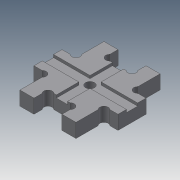
# Autodesk Inventor part: piece_1
Saved by Autodesk Inventor 2015 (Build 190159000, 159)
## iProperties
Created: 2017-11-05
Part Number: piece_1
Material: 一般
Document SubType Name: Modeling
Designer: tasuku
Density: 1 g/cm^3
Appearance: 既定
Author: tasuku
Autodesk Inventor part; units mm, degrees
ref_plane "YZ Plane" through (0, 0, 0) normal (1, 0, 0) x (0, 1, 0)
ref_plane "XZ Plane" through (0, 0, 0) normal (0, 1, 0) x (-1, 0, 0)
ref_plane "XY Plane" through (0, 0, 0) normal (0, 0, 1) x (1, 0, 0)
sketch "スケッチ1" plane through (0, 0, 0) normal (0, 0, 1) x (1, 0, 0)
  line L0 (-15, -15) -> (15, -15)
  line L1 (15, -15) -> (15, 15)
  line L2 (15, 15) -> (-15, 15)
  line L3 (-15, 15) -> (-15, -15)
  line L4 (-15, -15) -> (15, 15) construction
  line L5 (15, -15) -> (-15, 15) construction
  point P0 (0, 0)
  dimension "d2" = 30
  dimension "d3" = 30
  constraints: 12 end point, 2 midpoint, 2 parallel, 1 horizontal, 1 perpendicular
  measures "d2" distance of L1.end L2.end
  measures "d3" distance of L0.end L1.end
extrude "押し出し1" add sketch "スケッチ1" along normal blind 5
sketch "スケッチ2" plane through (0, 0, 5) normal (0, 0, 1) x (1, 0, 0)
  line L0 (-15, 15) -> (-10, 15)
  line L1 (-10, 15) -> (-10, 5)
  line L2 (-10, 5) -> (-15, 5)
  line L3 (-15, 5) -> (-15, 15)
  line L4 (-15, -15) -> (-10, -15)
  line L5 (-10, -15) -> (-10, -5)
  line L6 (-10, -5) -> (-15, -5)
  line L7 (-15, -5) -> (-15, -15)
  line L8 (15, 15) -> (-15, 15) projected
  line L9 (10, 15) -> (15, 15)
  line L10 (15, 15) -> (15, 5)
  line L11 (15, 5) -> (10, 5)
  line L12 (10, 5) -> (10, 15)
  line L13 (15, -15) -> (10, -15)
  line L14 (10, -15) -> (10, -5)
  line L15 (10, -5) -> (15, -5)
  line L16 (15, -5) -> (15, -15)
  line L17 (-5, 15) -> (5, 15)
  line L18 (5, 15) -> (5, 10)
  line L19 (5, 10) -> (-5, 10)
  line L20 (-5, 10) -> (-5, 15)
  line L21 (-15, -15) -> (15, -15) projected
  line L22 (-5, -15) -> (5, -15)
  line L23 (5, -15) -> (5, -10)
  line L24 (5, -10) -> (-5, -10)
  line L25 (-5, -10) -> (-5, -15)
  point P0 (0, 0)
  dimension "d6" = 10
  dimension "d7" = 10
  dimension "d8" = 5
  dimension "d9" = 10
  dimension "d10" = 5
  dimension "d11" = 5
  dimension "d12" = 10
  dimension "d13" = 10
  dimension "d14" = 5
  dimension "d15" = 5
  dimension "d16" = 5
  constraints: 48 end point, 12 parallel, 6 horizontal, 6 perpendicular, 6 point on line
  measures "d6" distance of L0.end L1.end
  measures "d7" distance of L4.end L5.end
  measures "d8" distance of L1.end L2.end
  measures "d9" distance of L11.end L9.start
  measures "d10" distance of L10.end L11.end
  measures "d11" distance of L14.end L15.end
  measures "d12" distance of L13.end L14.end
  measures "d13" distance of L18.end L19.end
  measures "d14" distance from line of point (0, 0) L20
  measures "d15" distance of L17.end L18.end
  measures "d16" distance of L22.end L23.end
extrude "押し出し2" cut sketch "スケッチ2" against normal blind 5
sketch "スケッチ4" plane through (0, 0, 5) normal (0, 0, 1) x (1, 0, 0)
  line L0 (-20.2222, 2) -> (20.2222, 2)
  line L1 (20.2222, 2) -> (20.2222, -2)
  line L2 (20.2222, -2) -> (-20.2222, -2)
  line L3 (-20.2222, -2) -> (-20.2222, 2)
  line L4 (-20.2222, 2) -> (20.2222, -2) construction
  line L5 (20.2222, 2) -> (-20.2222, -2) construction
  line L6 (-2, 16.5333) -> (2, 16.5333)
  line L7 (2, 16.5333) -> (2, -16.5333)
  line L8 (2, -16.5333) -> (-2, -16.5333)
  line L9 (-2, -16.5333) -> (-2, 16.5333)
  line L10 (-2, 16.5333) -> (2, -16.5333) construction
  line L11 (2, 16.5333) -> (-2, -16.5333) construction
  point P0 (0, 0)
  dimension "d19" = 4
  dimension "d20" = 4
  constraints: 24 end point, 4 midpoint, 4 parallel, 2 horizontal, 2 perpendicular
  measures "d19" distance of L6.start L6.end
  measures "d20" distance of L0.end L1.end
extrude "押し出し3" cut sketch "スケッチ4" against normal blind 1
sketch "スケッチ5" plane through (0, 0, 5) normal (0, 0, 1) x (1, 0, 0)
  circle A0 centre (0, 0) radius 1.6
  dimension "d23" = 3.2
  constraints: 1 centre point, 1 coincident
  measures "d23" diameter of A0
extrude "押し出し4" cut sketch "スケッチ5" against normal up to next
sketch "スケッチ7" plane through (0, 0, 5) normal (0, 0, 1) x (1, 0, 0)
  line L0 (-10, 5) -> (-11.0607, 6.0607) construction
  circle A0 centre (-11.0607, 6.0607) radius 1.5
  line L1 (-10, 5) -> (-15, 5) construction
  line L2 (-5, 10) -> (-3.8771, 10) construction
  line L3 (-2, 10) -> (-5, 10) projected
  line L4 (-5, 10) -> (-3.9393, 11.0607) construction
  circle A1 centre (-3.9393, 11.0607) radius 1.5
  line L5 (0, 0) -> (-3.2296, 0)
  line L6 (0, 0) -> (0, 2.4653)
  line L7 (10, 5) -> (11.0607, 6.0607) construction
  circle A2 centre (11.0607, 6.0607) radius 1.5
  line L8 (10, 5) -> (15, 5) construction
  line L9 (5, 10) -> (3.8771, 10) construction
  line L10 (2, 10) -> (5, 10)
  line L11 (5, 10) -> (3.9393, 11.0607) construction
  circle A3 centre (3.9393, 11.0607) radius 1.5
  line L12 (-10, -5) -> (-11.0607, -6.0607) construction
  circle A4 centre (-11.0607, -6.0607) radius 1.5
  line L13 (-10, -5) -> (-15, -5) construction
  line L14 (-5, -10) -> (-3.8771, -10) construction
  line L15 (-2, -10) -> (-5, -10)
  line L16 (-5, -10) -> (-3.9393, -11.0607) construction
  circle A5 centre (-3.9393, -11.0607) radius 1.5
  line L17 (10, -5) -> (11.0607, -6.0607) construction
  circle A6 centre (11.0607, -6.0607) radius 1.5
  line L18 (10, -5) -> (15, -5) construction
  line L19 (5, -10) -> (3.8771, -10) construction
  line L20 (2, -10) -> (5, -10)
  line L21 (5, -10) -> (3.9393, -11.0607) construction
  circle A7 centre (3.9393, -11.0607) radius 1.5
  dimension "d27" = 3
  dimension "d29" = 3
  dimension "d26" = 45
  dimension "d28" = 45
  constraints: 42 end point, 27 symmetric about line, 8 coincident, 6 horizontal, 4 point on line, 3 vertical, 24 other
  measures "d26" angle of L0 L1
  measures "d28" angle of L2 L4
extrude "押し出し5" cut sketch "スケッチ7" against normal up to next
